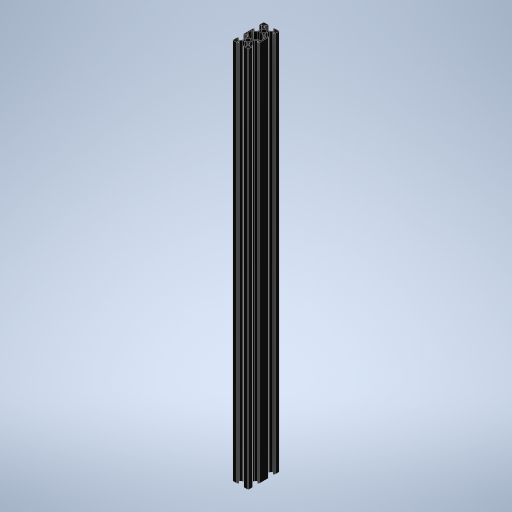
# Autodesk Inventor part: Perfil alumínio
Saved by Autodesk Inventor 2023 (Build 270158000, 158)
## iProperties
Created: 2023-04-15
Part Number: Perfil alumínio
Material: Aluminum 6061
Document SubType Name: Sheet Metal
Designer: Mateus PC
Density: 2.7 g/cm^3
Sheet Metal Rule: Default_mm
Appearance: Anodized - Black(edited)
Mass: 358.303 g
Surface Area: 1497.5 cm^2
Volume: 132.705 cm^3
Author: Mateus PC
Autodesk Inventor part; units mm, degrees
ref_plane "YZ Plane" through (0, 0, 0) normal (1, 0, 0) x (0, 1, 0)
ref_plane "XZ Plane" through (0, 0, 0) normal (0, 1, 0) x (-1, 0, 0)
ref_plane "XY Plane" through (0, 0, 0) normal (0, 0, 1) x (1, 0, 0)
sketch "Esboço2" plane through (0, 0, 0) normal (0, 1, 0) x (-1, 0, 0)
  line L0 (0.4, 0) -> (5.5515, 0)
  line L1 (7.4657, -1.5) -> (7.4657, -1.5)
  line L2 (6.5, -1.5) -> (4.9, -1.5)
  line L3 (4.5, -1.9) -> (4.5, -3.5)
  line L4 (4.6172, -3.7828) -> (6.3556, -5.5213)
  line L5 (6.7828, -0.8172) -> (6.2586, -0.2929)
  arc A0 (6.5, -1.5) -> (6.7828, -0.8172) centre (6.5, -1.1) ccw
  arc A1 (6.2586, -0.2929) -> (5.5515, 0) centre (5.5515, -1) ccw
  line L6 (0, -0.4) -> (0, -5.5489)
  line L7 (1.4976, -7.4655) -> (1.498, -7.4655)
  line L8 (1.4982, -6.4979) -> (1.4987, -4.8999)
  line L9 (1.8987, -4.5) -> (3.3343, -4.5)
  line L10 (3.6172, -4.6172) -> (5.5213, -6.5213)
  line L11 (0.8153, -6.7805) -> (0.2929, -6.256)
  arc A2 (0.8153, -6.7805) -> (1.4982, -6.4979) centre (1.0982, -6.4978) ccw
  arc A3 (0, -5.5489) -> (0.2929, -6.256) centre (1, -5.5489) ccw
  arc A4 (0.2929, -13.7414) -> (0, -14.4485) centre (1, -14.4485) ccw
  line L12 (1.4963, -13.5004) -> (1.4959, -15.0999)
  line L13 (0.8135, -13.2174) -> (0.2929, -13.7414)
  arc A5 (1.4963, -13.5004) -> (0.8135, -13.2174) centre (1.0963, -13.5003) ccw
  line L14 (1.4961, -12.5304) -> (1.4966, -12.5304)
  line L15 (1.8959, -15.5) -> (3.3343, -15.5)
  line L16 (3.6172, -15.3828) -> (5.5213, -13.4787)
  line L17 (0, -20) -> (0, -14.4485)
  line L18 (19.6, 0) -> (14.4485, 0)
  line L19 (12.5343, -1.5) -> (12.5343, -1.5)
  line L20 (13.5, -1.5) -> (15.1, -1.5)
  line L21 (15.5, -1.9) -> (15.5, -3.3343)
  line L22 (15.3828, -3.6172) -> (13.4787, -5.5213)
  line L23 (13.2172, -0.8172) -> (13.7414, -0.2929)
  arc A6 (13.2172, -0.8172) -> (13.5, -1.5) centre (13.5, -1.1) ccw
  arc A7 (14.4485, 0) -> (13.7414, -0.2929) centre (14.4485, -1) ccw
  arc A8 (19.7071, -6.2586) -> (20, -5.5515) centre (19, -5.5515) ccw
  line L24 (18.5, -6.5) -> (18.5, -4.9)
  line L25 (19.1828, -6.7828) -> (19.7071, -6.2586)
  arc A9 (18.5, -6.5) -> (19.1828, -6.7828) centre (18.9, -6.5) ccw
  line L26 (18.5, -7.4657) -> (18.5, -7.4657)
  line L27 (18.1, -4.5) -> (16.6657, -4.5)
  line L28 (16.3828, -4.6172) -> (14.4787, -6.5213)
  line L29 (20, -0.4) -> (20, -5.5515)
  line L30 (18.5, -13.5) -> (18.5, -15.1)
  line L31 (18.1, -15.5) -> (16.6657, -15.5)
  line L32 (16.3828, -15.3828) -> (14.4787, -13.4787)
  line L33 (20, -20) -> (20, -14.4485)
  arc A10 (19.1828, -13.2172) -> (18.5, -13.5) centre (18.9, -13.5) ccw
  line L34 (18.5, -12.5343) -> (18.5, -12.5343)
  line L35 (19.1828, -13.2172) -> (19.7071, -13.7414)
  arc A11 (20, -14.4485) -> (19.7071, -13.7414) centre (19, -14.4485) ccw
  line L36 (8.477, -6.4) -> (11.3574, -6.4)
  line L37 (13.6, -8.6426) -> (13.6, -11.3574)
  line L38 (11.3574, -13.6) -> (8.6426, -13.6)
  line L39 (6.4, -11.3574) -> (6.4, -8.6426)
  line L40 (18.5, -20) -> (18.5, -17.4)
  line L41 (13.4787, -14.4787) -> (15.8828, -16.8828)
  line L42 (16.1657, -17) -> (18.1, -17)
  line L43 (6.5213, -14.4787) -> (4.1172, -16.8828)
  line L44 (3.8343, -17) -> (1.9, -17)
  line L45 (1.5, -17.4) -> (1.5, -20)
  line L46 (0.4, -40.0001) -> (5.5406, -40.0001)
  line L47 (7.4548, -38.5001) -> (7.4548, -38.5001)
  line L48 (6.4892, -38.5001) -> (4.8892, -38.5001)
  line L49 (4.4892, -38.1001) -> (4.4892, -36.6658)
  line L50 (4.6063, -36.383) -> (6.5105, -34.4788)
  line L51 (6.772, -39.183) -> (6.2477, -39.7072)
  arc A12 (6.772, -39.183) -> (6.4892, -38.5001) centre (6.4892, -38.9001) ccw
  arc A13 (5.5406, -40.0001) -> (6.2477, -39.7072) centre (5.5406, -39.0001) ccw
  arc A14 (0.2929, -33.7414) -> (0, -34.4485) centre (1, -34.4485) ccw
  line L52 (1.5, -33.5) -> (1.5, -35.1)
  line L53 (0.8172, -33.2172) -> (0.2929, -33.7414)
  arc A15 (1.5, -33.5) -> (0.8172, -33.2172) centre (1.1, -33.5) ccw
  line L54 (1.5, -32.5343) -> (1.5, -32.5343)
  line L55 (1.9, -35.5) -> (3.3343, -35.5)
  line L56 (3.6172, -35.3828) -> (5.5213, -33.4787)
  line L57 (0, -39.6001) -> (0, -34.4485)
  line L58 (1.5, -26.5) -> (1.5, -24.9)
  line L59 (1.9, -24.5) -> (3.3343, -24.5)
  line L60 (3.6172, -24.6172) -> (5.5213, -26.5213)
  line L61 (0, -20) -> (0, -25.5515)
  arc A16 (0.8172, -26.7828) -> (1.5, -26.5) centre (1.1, -26.5) ccw
  line L62 (1.5, -27.4657) -> (1.5, -27.4657)
  line L63 (0.8172, -26.7828) -> (0.2929, -26.2586)
  arc A17 (0, -25.5515) -> (0.2929, -26.2586) centre (1, -25.5515) ccw
  line L64 (19.6, -40.0001) -> (14.4377, -40.0001)
  line L65 (12.5235, -38.5001) -> (12.5235, -38.5001)
  line L66 (13.4892, -38.5001) -> (15.0892, -38.5001)
  line L67 (15.4892, -38.1001) -> (15.4892, -36.6658)
  line L68 (15.372, -36.383) -> (13.4678, -34.4788)
  line L69 (13.2063, -39.183) -> (13.7306, -39.7072)
  arc A18 (13.4892, -38.5001) -> (13.2063, -39.183) centre (13.4892, -38.9001) ccw
  line L70 (18.5, -27.4657) -> (18.5, -27.4657)
  arc A19 (18.5, -26.5) -> (19.1828, -26.7828) centre (18.9, -26.5) ccw
  line L71 (19.1828, -26.7828) -> (19.7071, -26.2586)
  arc A20 (19.7071, -26.2586) -> (20, -25.5515) centre (19, -25.5515) ccw
  arc A21 (13.7306, -39.7072) -> (14.4377, -40.0001) centre (14.4377, -39.0001) ccw
  line L72 (18.5, -32.5343) -> (18.5, -32.5343)
  arc A22 (19.1828, -33.2172) -> (18.5, -33.5) centre (18.9, -33.5) ccw
  line L73 (19.1828, -33.2172) -> (19.7071, -33.7414)
  arc A23 (20, -34.4485) -> (19.7071, -33.7414) centre (19, -34.4485) ccw
  line L74 (16.5, -35.5) -> (14.4787, -33.4787)
  line L75 (18.1, -35.5) -> (16.5, -35.5)
  line L76 (20, -39.6001) -> (20, -34.4485)
  line L77 (18.5, -33.5) -> (18.5, -35.1)
  line L78 (18.5, -26.5) -> (18.5, -24.9)
  line L79 (18.1, -24.5) -> (16.6657, -24.5)
  line L80 (20, -20) -> (20, -25.5515)
  line L81 (16.3828, -24.6172) -> (14.4787, -26.5213)
  line L82 (8.6318, -33.6001) -> (11.3465, -33.6001)
  line L83 (13.6, -31.3574) -> (13.6, -28.6426)
  line L84 (11.3574, -26.4) -> (8.6426, -26.4)
  line L85 (6.4, -28.6426) -> (6.4, -31.3574)
  line L86 (18.5, -20) -> (18.5, -22.6)
  line L87 (13.4787, -25.5213) -> (15.8828, -23.1172)
  line L88 (16.1657, -23) -> (18.1, -23)
  line L89 (6.5213, -25.5213) -> (4.1172, -23.1172)
  line L90 (3.8343, -23) -> (1.9, -23)
  line L91 (1.5, -22.6) -> (1.5, -20)
  arc A24 (11.3574, -6.4) -> (13.4787, -5.5213) centre (11.3574, -3.4) ccw
  arc A25 (6.3556, -5.5213) -> (8.477, -6.4) centre (8.477, -3.4) ccw
  arc A26 (6.4, -8.6426) -> (5.5213, -6.5213) centre (3.4, -8.6426) ccw
  arc A27 (5.5213, -13.4787) -> (6.4, -11.3574) centre (3.4, -11.3574) ccw
  arc A28 (13.6, -11.3574) -> (14.4787, -13.4787) centre (16.6, -11.3574) ccw
  arc A29 (14.4787, -6.5213) -> (13.6, -8.6426) centre (16.6, -8.6426) ccw
  arc A30 (13.4787, -14.4787) -> (11.3574, -13.6) centre (11.3574, -16.6) ccw
  arc A31 (8.6426, -13.6) -> (6.5213, -14.4787) centre (8.6426, -16.6) ccw
  arc A32 (11.3574, -26.4) -> (13.4787, -25.5213) centre (11.3574, -23.4) ccw
  arc A33 (6.4, -28.6426) -> (5.5213, -26.5213) centre (3.4, -28.6426) ccw
  arc A34 (6.5213, -25.5213) -> (8.6426, -26.4) centre (8.6426, -23.4) ccw
  arc A35 (5.5213, -33.4787) -> (6.4, -31.3574) centre (3.4, -31.3574) ccw
  arc A36 (8.6318, -33.6001) -> (6.5105, -34.4788) centre (8.6318, -36.6001) ccw
  arc A37 (13.4678, -34.4788) -> (11.3465, -33.6001) centre (11.3465, -36.6001) ccw
  arc A38 (13.6, -31.3574) -> (14.4787, -33.4787) centre (16.6, -31.3574) ccw
  arc A39 (14.4787, -26.5213) -> (13.6, -28.6426) centre (16.6, -28.6426) ccw
  circle A40 centre (10, -10) radius 2.5
  circle A41 centre (10, -30) radius 2.5
  arc A42 (18.5, -17.4) -> (18.1, -17) centre (18.1, -17.4) ccw
  arc A43 (18.1, -23) -> (18.5, -22.6) centre (18.1, -22.6) ccw
  arc A44 (1.5, -22.6) -> (1.9, -23) centre (1.9, -22.6) ccw
  arc A45 (1.9, -17) -> (1.5, -17.4) centre (1.9, -17.4) ccw
  arc A46 (4.1172, -23.1172) -> (3.8343, -23) centre (3.8343, -23.4) ccw
  arc A47 (3.8343, -17) -> (4.1172, -16.8828) centre (3.8343, -16.6) ccw
  arc A48 (15.8828, -16.8828) -> (16.1657, -17) centre (16.1657, -16.6) ccw
  arc A49 (16.6657, -24.5) -> (16.3828, -24.6172) centre (16.6657, -24.9) ccw
  arc A50 (16.1657, -23) -> (15.8828, -23.1172) centre (16.1657, -23.4) ccw
  arc A51 (3.6172, -24.6172) -> (3.3343, -24.5) centre (3.3343, -24.9) ccw
  arc A52 (1.9, -24.5) -> (1.5, -24.9) centre (1.9, -24.9) ccw
  arc A53 (1.5, -35.1) -> (1.9, -35.5) centre (1.9, -35.1) ccw
  arc A54 (3.3343, -35.5) -> (3.6172, -35.3828) centre (3.3343, -35.1) ccw
  arc A55 (4.6063, -36.383) -> (4.4892, -36.6658) centre (4.8892, -36.6658) ccw
  arc A56 (4.4892, -38.1001) -> (4.8892, -38.5001) centre (4.8892, -38.1001) ccw
  arc A57 (15.4892, -36.6658) -> (15.372, -36.383) centre (15.0892, -36.6658) ccw
  arc A58 (15.0892, -38.5001) -> (15.4892, -38.1001) centre (15.0892, -38.1001) ccw
  arc A59 (19.6, -40.0001) -> (20, -39.6001) centre (19.6, -39.6001) ccw
  arc A60 (18.1, -35.5) -> (18.5, -35.1) centre (18.1, -35.1) ccw
  arc A61 (18.5, -24.9) -> (18.1, -24.5) centre (18.1, -24.9) ccw
  arc A62 (18.1, -15.5) -> (18.5, -15.1) centre (18.1, -15.1) ccw
  arc A63 (16.3828, -15.3828) -> (16.6657, -15.5) centre (16.6657, -15.1) ccw
  arc A64 (16.6657, -4.5) -> (16.3828, -4.6172) centre (16.6657, -4.9) ccw
  arc A65 (18.5, -4.9) -> (18.1, -4.5) centre (18.1, -4.9) ccw
  arc A66 (20, -0.4) -> (19.6, 0) centre (19.6, -0.4) ccw
  arc A67 (15.5, -1.9) -> (15.1, -1.5) centre (15.1, -1.9) ccw
  arc A68 (15.3828, -3.6172) -> (15.5, -3.3343) centre (15.1, -3.3343) ccw
  arc A69 (4.5, -3.5) -> (4.6172, -3.7828) centre (4.9, -3.5) ccw
  arc A70 (4.9, -1.5) -> (4.5, -1.9) centre (4.9, -1.9) ccw
  arc A71 (0.4, 0) -> (0, -0.4) centre (0.4, -0.4) ccw
  arc A72 (1.8987, -4.5) -> (1.4987, -4.8999) centre (1.8987, -4.9) ccw
  arc A73 (3.6172, -4.6172) -> (3.3343, -4.5) centre (3.3343, -4.9) ccw
  arc A74 (3.3343, -15.5) -> (3.6172, -15.3828) centre (3.3343, -15.1) ccw
  arc A75 (1.4959, -15.0999) -> (1.8959, -15.5) centre (1.8959, -15.1) ccw
  arc A76 (0, -39.6001) -> (0.4, -40.0001) centre (0.4, -39.6001) ccw
  point P0 (0, 0)
  point P1 (7.4657, 0)
  point P2 (4.5, -1.5)
  point P3 (7.2343, -6.4)
  point P4 (0, -7.4626)
  point P5 (6.4, -7.4)
  point P6 (7.4, -13.6)
  point P7 (0, -12.5353)
  point P8 (6.4, -12.6)
  point P9 (20, 0)
  point P10 (12.5343, 0)
  point P11 (20, -10)
  point P12 (20, -7.4657)
  point P13 (12.6, -13.6)
  point P14 (20, -12.5343)
  point P15 (2.9757, 0)
  point P16 (18.5, -17)
  point P17 (7.4548, -40.0001)
  point P18 (0, -30)
  point P19 (0, -32.5343)
  point P20 (0, -27.4657)
  point P21 (12.5235, -40.0001)
  point P22 (20, -30)
  point P23 (20, -27.4657)
  point P24 (20, -32.5343)
  point P25 (2.7757, -40)
  dimension "d137" = 4.5
  dimension "d138" = 45
  dimension "d139" = 6.4
  dimension "d141" = 1.5
  dimension "d142" = 1.5
  dimension "d145" = 0.4
  dimension "d146" = 6.5
  dimension "d147" = 45
  dimension "d148" = 1
  dimension "d151" = 20
  dimension "d152" = 20
  dimension "d153" = 5.2
  dimension "d154" = 7.4
  dimension "d155" = 13.6
  dimension "d156" = 3
  dimension "d157" = 135
  dimension "d158" = 3
  dimension "d159" = 5
  dimension "d160" = 5
  dimension "d161" = 0.4
  constraints: 182 end point, 150 point on circle, 105 tangent, 77 centre point, 65 point on line, 49 equal radius, 7 collinear, 6 horizontal, 6 perpendicular, 4 vertical, 1 midpoint, 5 other
  measures "d137" horizontal distance of point (0, 0) point (4.5, -1.5)
  measures "d138" angle of L0 L4
  measures "d139" vertical distance of point (7.466, 0) point (7.234, -6.4)
  measures "d141" distance of point (7.466, 0) L1.end
  measures "d142" distance of L1.start point (7.466, 0)
  measures "d145" radius of A0
  measures "d146" horizontal distance of point (0, 0) A0.centre
  measures "d147" angle of L2 L5
  measures "d148" radius of A1
  measures "d151" distance of point (0, 0) point (20, 0)
  measures "d152" distance of L33.start point (20, 0)
  measures "d153" distance of point (12.6, -13.6) point (7.4, -13.6)
  measures "d154" distance from line of L6 point (7.4, -13.6)
  measures "d155" vertical distance of point (2.976, 0) point (7.4, -13.6)
  measures "d156" distance of L40.start point (18.5, -17)
  measures "d157" angle of L38 L41
  measures "d158" radius of A24
  measures "d159" diameter of A40
  measures "d160" diameter of A41
  measures "d161" radius of A42
extrude "Extrusão1" add sketch "Esboço2" along normal blind 490
equation "\"Raio_vergadura\" = Espessura"
equation "\"Largura_alívio_de_vergadura\" = Espessura"
equation "\"Profundidade_alívio_de_vergadura\" = 0.5 * Espessura"
equation "\"Tamanho_alívio_de_dobra\" = 4 * Espessura"
equation "\"Remanescente_mínimo\" = 2 * Espessura"
equation "\"Raiodetransição\" = Raio_vergadura"
equation "\"Tamanho_de_raio_de_Jacobi\" = Raio_vergadura"
equation "\"TamanhoFolga\" = Espessura"
equation "\"Espessura\" = 0.5"
